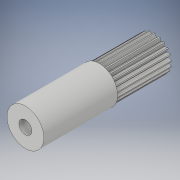
# Autodesk Inventor part: Part10
Saved by Autodesk Inventor 2017 SP1 (Build 210196100, 196)
## iProperties
Created: 2017-05-14
Part Number: Part10
Material: Generic
Document SubType Name: Modeling
Designer: Zach
Density: 1 g/cm^3
Appearance: Default
Author: Zach
Autodesk Inventor part; units mm, degrees
ref_plane "YZ Plane" through (0, 0, 0) normal (1, 0, 0) x (0, 1, 0)
ref_plane "XZ Plane" through (0, 0, 0) normal (0, 1, 0) x (-1, 0, 0)
ref_plane "XY Plane" through (0, 0, 0) normal (0, 0, 1) x (1, 0, 0)
sketch "Sketch1" plane through (0, 0, 0) normal (0, 0, 1) x (1, 0, 0)
  circle A0 centre (0, 0) radius 10
  dimension "d0" = 20
  constraints: 1 centre point, 1 coincident
  measures "d0" diameter of A0
extrude "Extrusion1" add sketch "Sketch1" along normal blind 40
sketch "Sketch2" plane through (0, 0, 0) normal (0, 0, -1) x (-1, 0, 0)
  circle A0 centre (0, 0) radius 7.5
  dimension "d3" = 15
  constraints: 1 centre point, 1 coincident
  measures "d3" diameter of A0
extrude "Extrusion2" add sketch "Sketch2" along normal blind 30
sketch "Sketch3" plane through (0, 0, -30) normal (0, 0, -1) x (-1, 0, 0)
  circle A0 centre (0, 0) radius 3.5
  dimension "d6" = 7
  constraints: 1 centre point, 1 coincident
  measures "d6" diameter of A0
extrude "Extrusion3" cut sketch "Sketch3" against normal through all
sketch "Sketch4" plane through (0, 0, 0) normal (0, 0, -1) x (-1, 0, 0)
  line L0 (0, 0) -> (0, 11.2895) construction
  arc A0 (1, 7.433) -> (-1, 7.433) centre (0, 0) ccw
  line L1 (-1, 7.433) -> (0, 10) construction
  line L2 (1, 7.433) -> (0, 10) construction
  line L3 (-1, 7.433) -> (-0.274, 9.2966)
  line L4 (-0.274, 9.2966) -> (0.274, 9.2966)
  line L5 (1, 7.433) -> (0.274, 9.2966)
  arc A1 (-1.2354, 7.3976) -> (-3.1465, 6.8081) centre (0, 0) ccw
  line L6 (-3.0021, 8.8028) -> (-2.4784, 8.9644)
  line L7 (-3.1465, 6.8081) -> (-2.9476, 9.5557) construction
  line L8 (-3.1465, 6.8081) -> (-3.0021, 8.8028)
  line L9 (-1.2354, 7.3976) -> (-2.9476, 9.5557) construction
  line L10 (-1.2354, 7.3976) -> (-2.4784, 8.9644)
  arc A2 (-3.3609, 6.7048) -> (-5.0134, 5.5781) centre (0, 0) ccw
  line L11 (-5.4634, 7.5269) -> (-5.0106, 7.8356)
  line L12 (-5.0134, 5.5781) -> (-5.6332, 8.2624) construction
  line L13 (-5.0134, 5.5781) -> (-5.4634, 7.5269)
  line L14 (-3.3609, 6.7048) -> (-5.6332, 8.2624) construction
  line L15 (-3.3609, 6.7048) -> (-5.0106, 7.8356)
  arc A3 (-5.1879, 5.4163) -> (-6.4349, 3.8526) centre (0, 0) ccw
  line L16 (-7.4392, 5.5821) -> (-7.0975, 6.0106)
  line L17 (-6.4349, 3.8526) -> (-7.8183, 6.2349) construction
  line L18 (-6.4349, 3.8526) -> (-7.4392, 5.5821)
  line L19 (-5.1879, 5.4163) -> (-7.8183, 6.2349) construction
  line L20 (-5.1879, 5.4163) -> (-7.0975, 6.0106)
  arc A4 (-6.5539, 3.6465) -> (-7.2846, 1.7847) centre (0, 0) ccw
  line L21 (-8.7541, 3.1414) -> (-8.5539, 3.6515)
  line L22 (-7.2846, 1.7847) -> (-9.3087, 3.6534) construction
  line L23 (-7.2846, 1.7847) -> (-8.7541, 3.1414)
  line L24 (-6.5539, 3.6465) -> (-9.3087, 3.6534) construction
  line L25 (-6.5539, 3.6465) -> (-8.5539, 3.6515)
  arc A5 (-7.3375, 1.5527) -> (-7.487, -0.4417) centre (0, 0) ccw
  line L26 (-9.2911, 0.4215) -> (-9.2501, 0.968)
  line L27 (-7.487, -0.4417) -> (-9.972, 0.7473) construction
  line L28 (-7.487, -0.4417) -> (-9.2911, 0.4215)
  line L29 (-7.3375, 1.5527) -> (-9.972, 0.7473) construction
  line L30 (-7.3375, 1.5527) -> (-9.2501, 0.968)
  arc A6 (-7.4692, -0.6791) -> (-7.0242, -2.6289) centre (0, 0) ccw
  line L31 (-9.0026, -2.3358) -> (-9.1245, -1.8015)
  line L32 (-7.0242, -2.6289) -> (-9.7493, -2.2252) construction
  line L33 (-7.0242, -2.6289) -> (-9.0026, -2.3358)
  line L34 (-7.4692, -0.6791) -> (-9.7493, -2.2252) construction
  line L35 (-7.4692, -0.6791) -> (-9.1245, -1.8015)
  arc A7 (-6.9372, -2.8505) -> (-5.9372, -4.5825) centre (0, 0) ccw
  line L36 (-7.9141, -4.8856) -> (-8.1881, -4.411)
  line L37 (-5.9372, -4.5825) -> (-8.6603, -5) construction
  line L38 (-5.9372, -4.5825) -> (-7.9141, -4.8856)
  line L39 (-6.9372, -2.8505) -> (-8.6603, -5) construction
  line L40 (-6.9372, -2.8505) -> (-8.1881, -4.411)
  arc A8 (-5.7888, -4.7686) -> (-4.3227, -6.129) centre (0, 0) ccw
  line L41 (-6.1224, -7.0013) -> (-6.5242, -6.6285)
  line L42 (-4.3227, -6.129) -> (-6.8017, -7.3305) construction
  line L43 (-4.3227, -6.129) -> (-6.1224, -7.0013)
  line L44 (-5.7888, -4.7686) -> (-6.8017, -7.3305) construction
  line L45 (-5.7888, -4.7686) -> (-6.5242, -6.6285)
  arc A9 (-4.126, -6.263) -> (-2.3241, -7.1308) centre (0, 0) ccw
  line L46 (-3.7868, -8.4949) -> (-4.2805, -8.2571)
  line L47 (-2.3241, -7.1308) -> (-4.3388, -9.0097) construction
  line L48 (-2.3241, -7.1308) -> (-3.7868, -8.4949)
  line L49 (-4.126, -6.263) -> (-4.3388, -9.0097) construction
  line L50 (-4.126, -6.263) -> (-4.2805, -8.2571)
  arc A10 (-2.0967, -7.201) -> (-0.119, -7.4991) centre (0, 0) ccw
  line L51 (-1.1146, -9.2336) -> (-1.6565, -9.1519)
  line L52 (-0.119, -7.4991) -> (-1.4904, -9.8883) construction
  line L53 (-0.119, -7.4991) -> (-1.1146, -9.2336)
  line L54 (-2.0967, -7.201) -> (-1.4904, -9.8883) construction
  line L55 (-2.0967, -7.201) -> (-1.6565, -9.1519)
  arc A11 (0.119, -7.4991) -> (2.0967, -7.201) centre (0, 0) ccw
  line L56 (1.6565, -9.1519) -> (1.1146, -9.2336)
  line L57 (2.0967, -7.201) -> (1.4904, -9.8883) construction
  line L58 (2.0967, -7.201) -> (1.6565, -9.1519)
  line L59 (0.119, -7.4991) -> (1.4904, -9.8883) construction
  line L60 (0.119, -7.4991) -> (1.1146, -9.2336)
  arc A12 (2.3241, -7.1308) -> (4.126, -6.263) centre (0, 0) ccw
  line L61 (4.2805, -8.2571) -> (3.7868, -8.4949)
  line L62 (4.126, -6.263) -> (4.3388, -9.0097) construction
  line L63 (4.126, -6.263) -> (4.2805, -8.2571)
  line L64 (2.3241, -7.1308) -> (4.3388, -9.0097) construction
  line L65 (2.3241, -7.1308) -> (3.7868, -8.4949)
  arc A13 (4.3227, -6.129) -> (5.7888, -4.7686) centre (0, 0) ccw
  line L66 (6.5242, -6.6285) -> (6.1224, -7.0013)
  line L67 (5.7888, -4.7686) -> (6.8017, -7.3305) construction
  line L68 (5.7888, -4.7686) -> (6.5242, -6.6285)
  line L69 (4.3227, -6.129) -> (6.8017, -7.3305) construction
  line L70 (4.3227, -6.129) -> (6.1224, -7.0013)
  arc A14 (5.9372, -4.5825) -> (6.9372, -2.8505) centre (0, 0) ccw
  line L71 (8.1881, -4.411) -> (7.9141, -4.8856)
  line L72 (6.9372, -2.8505) -> (8.6603, -5) construction
  line L73 (6.9372, -2.8505) -> (8.1881, -4.411)
  line L74 (5.9372, -4.5825) -> (8.6603, -5) construction
  line L75 (5.9372, -4.5825) -> (7.9141, -4.8856)
  arc A15 (7.0242, -2.6289) -> (7.4692, -0.6791) centre (0, 0) ccw
  line L76 (9.1245, -1.8015) -> (9.0026, -2.3358)
  line L77 (7.4692, -0.6791) -> (9.7493, -2.2252) construction
  line L78 (7.4692, -0.6791) -> (9.1245, -1.8015)
  line L79 (7.0242, -2.6289) -> (9.7493, -2.2252) construction
  line L80 (7.0242, -2.6289) -> (9.0026, -2.3358)
  arc A16 (7.487, -0.4417) -> (7.3375, 1.5527) centre (0, 0) ccw
  line L81 (9.2501, 0.968) -> (9.2911, 0.4215)
  line L82 (7.3375, 1.5527) -> (9.972, 0.7473) construction
  line L83 (7.3375, 1.5527) -> (9.2501, 0.968)
  line L84 (7.487, -0.4417) -> (9.972, 0.7473) construction
  line L85 (7.487, -0.4417) -> (9.2911, 0.4215)
  arc A17 (7.2846, 1.7847) -> (6.5539, 3.6465) centre (0, 0) ccw
  line L86 (8.5539, 3.6515) -> (8.7541, 3.1414)
  line L87 (6.5539, 3.6465) -> (9.3087, 3.6534) construction
  line L88 (6.5539, 3.6465) -> (8.5539, 3.6515)
  line L89 (7.2846, 1.7847) -> (9.3087, 3.6534) construction
  line L90 (7.2846, 1.7847) -> (8.7541, 3.1414)
  arc A18 (6.4349, 3.8526) -> (5.1879, 5.4163) centre (0, 0) ccw
  line L91 (7.0975, 6.0106) -> (7.4392, 5.5821)
  line L92 (5.1879, 5.4163) -> (7.8183, 6.2349) construction
  line L93 (5.1879, 5.4163) -> (7.0975, 6.0106)
  line L94 (6.4349, 3.8526) -> (7.8183, 6.2349) construction
  line L95 (6.4349, 3.8526) -> (7.4392, 5.5821)
  arc A19 (5.0134, 5.5781) -> (3.3609, 6.7048) centre (0, 0) ccw
  line L96 (5.0106, 7.8356) -> (5.4634, 7.5269)
  line L97 (3.3609, 6.7048) -> (5.6332, 8.2624) construction
  line L98 (3.3609, 6.7048) -> (5.0106, 7.8356)
  line L99 (5.0134, 5.5781) -> (5.6332, 8.2624) construction
  line L100 (5.0134, 5.5781) -> (5.4634, 7.5269)
  arc A20 (3.1465, 6.8081) -> (1.2354, 7.3976) centre (0, 0) ccw
  line L101 (2.4784, 8.9644) -> (3.0021, 8.8028)
  line L102 (1.2354, 7.3976) -> (2.9476, 9.5557) construction
  line L103 (1.2354, 7.3976) -> (2.4784, 8.9644)
  line L104 (3.1465, 6.8081) -> (2.9476, 9.5557) construction
  line L105 (3.1465, 6.8081) -> (3.0021, 8.8028)
  circle A21 centre (0, 0) radius 7.5 projected
  dimension "d9" = 10
  dimension "d12" = 7.5
  dimension "d19" = 2
  dimension "d21" = 2
  dimension "d24" = 360
  constraints: 212 end point, 43 point on line, 42 point on circle, 21 centre point, 2 coincident, 1 collinear, 1 concentric, 1 horizontal, 1 symmetric about line, 1 vertical, 251 other
  measures "d9" distance of L0.start L1.end
  measures "d12" radius of A0
  measures "d19" distance of L1.start L3.end
  measures "d21" distance of L2.start L1.start
extrude "Extrusion4" add sketch "Sketch4" along normal blind 30 contours A0 L3 L4 L5 | L103 L101 L105 A20 | A1 L8 L6 L10 | L98 L96 L100 A19 | A2 L13 L11 L15 | L93 L91 L95 A18 | A3 L18 L16 L20 | L88 L86 L90 A17 | A4 L23 L21 L25 | L83 L81 L85 A16 | A5 L28 L26 L30 | A6 L33 L31 L35 | L78 L76 L80 A15 | A7 L38 L36 L40 | L73 L71 L75 A14 | A8 L43 L41 L45 | L68 L66 L70 A13 | A9 L48 L46 L50 | L63 L61 L65 A12 | A10 L53 L51 L55 | L58 L56 L60 A11
body "Solid1"
